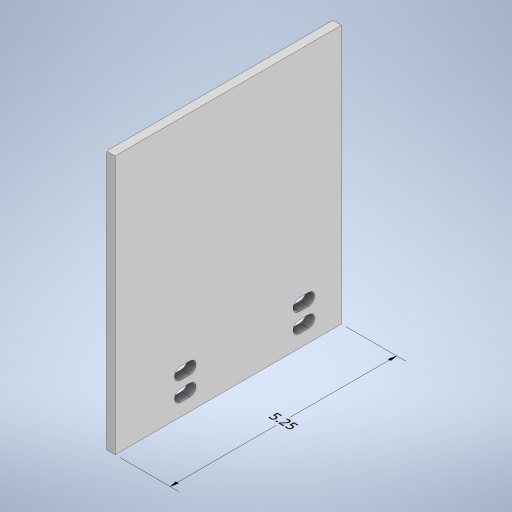
# Autodesk Inventor part: HalfFrontWall
Saved by Autodesk Inventor 2024.3 (Build 283343010, 343A)
## iProperties
Created: 2025-04-11
Part Number: HalfFrontWall
Material: Generic
Document SubType Name: Modeling
Designer: Vincent Larson
Density: 1 g/cm^3
Appearance: Default
Author: Vincent Larson
Autodesk Inventor part; units mm, degrees
ref_plane "YZ Plane" through (0, 0, 0) normal (1, 0, 0) x (0, 1, 0)
ref_plane "XZ Plane" through (0, 0, 0) normal (0, 1, 0) x (-1, 0, 0)
ref_plane "XY Plane" through (0, 0, 0) normal (0, 0, 1) x (1, 0, 0)
sketch "Sketch1" plane through (0, 0, 0) normal (0, 0, 1) x (1, 0, 0)
  point P0 (0, 0)
sketch "Sketch2" plane through (0, 0, 0) normal (1, 0, 0) x (0, 1, 0)
  line L0 (0, 0) -> (-152.4, 0)
  line L1 (-152.4, 0) -> (-152.4, -133.35)
  line L2 (-152.4, -133.35) -> (0, -133.35)
  line L3 (0, -133.35) -> (0, 0)
  dimension "d0" = 152.4
  dimension "d1" = 133.35
  constraints: 8 end point, 2 parallel, 1 horizontal, 1 perpendicular
  measures "d0" distance of L2.end L1.end
  measures "d1" distance of L1.end L0.end
extrude "Extrusion1" add sketch "Sketch2" along normal blind 5.08
sketch "Sketch6" plane through (5.08, 0, 0) normal (1, 0, 0) x (0, 0, -1)
  line L0 (0, -152.4) -> (133.35, -152.4) projected
  line L1 (133.35, -152.4) -> (133.35, 0) projected
  line L2 (0, 0) -> (0, -152.4) projected
  line L3 (41.275, -130.048) -> (47.625, -130.048)
  line L4 (47.625, -130.048) -> (41.275, -130.048)
  line L5 (41.275, -130.048) -> (34.925, -130.048)
  line L6 (34.925, -130.048) -> (47.625, -130.048) construction
  line L7 (38.4175, -133.5405) -> (44.1325, -133.5405)
  line L8 (44.1325, -126.5555) -> (38.4175, -126.5555)
  arc A0 (38.4175, -126.5555) -> (38.4175, -133.5405) centre (38.4175, -130.048) ccw
  arc A1 (44.1325, -133.5405) -> (44.1325, -126.5555) centre (44.1325, -130.048) ccw
  line L9 (111.125, -130.048) -> (117.475, -130.048)
  line L10 (117.475, -130.048) -> (111.125, -130.048)
  line L11 (111.125, -130.048) -> (104.775, -130.048)
  line L12 (104.775, -130.048) -> (117.475, -130.048) construction
  line L13 (108.2675, -133.5405) -> (113.9825, -133.5405)
  line L14 (113.9825, -126.5555) -> (108.2675, -126.5555)
  arc A2 (108.2675, -126.5555) -> (108.2675, -133.5405) centre (108.2675, -130.048) ccw
  arc A3 (113.9825, -133.5405) -> (113.9825, -126.5555) centre (113.9825, -130.048) ccw
  line L15 (41.275, -141.351) -> (47.625, -141.351)
  line L16 (47.625, -141.351) -> (41.275, -141.351)
  line L17 (41.275, -141.351) -> (34.925, -141.351)
  line L18 (34.925, -141.351) -> (47.625, -141.351) construction
  line L19 (38.4175, -144.8435) -> (44.1325, -144.8435)
  line L20 (44.1325, -137.8585) -> (38.4175, -137.8585)
  arc A4 (38.4175, -137.8585) -> (38.4175, -144.8435) centre (38.4175, -141.351) ccw
  arc A5 (44.1325, -144.8435) -> (44.1325, -137.8585) centre (44.1325, -141.351) ccw
  line L21 (111.125, -141.351) -> (117.475, -141.351)
  line L22 (111.125, -141.351) -> (104.775, -141.351)
  line L23 (104.775, -141.351) -> (117.475, -141.351) construction
  line L24 (108.2675, -144.8435) -> (113.9825, -144.8435)
  line L25 (113.9825, -137.8585) -> (108.2675, -137.8585)
  arc A6 (108.2675, -137.8585) -> (108.2675, -144.8435) centre (108.2675, -141.351) ccw
  arc A7 (113.9825, -144.8435) -> (113.9825, -137.8585) centre (113.9825, -141.351) ccw
  dimension "d28" = 6.35
  dimension "d30" = 6.985
  dimension "d31" = 6.35
  dimension "d32" = 6.35
  dimension "d33" = 6.985
  dimension "d34" = 6.35
  dimension "d35" = 6.35
  dimension "d36" = 6.985
  dimension "d37" = 6.35
  dimension "d38" = 6.35
  dimension "d39" = 6.985
  constraints: 54 end point, 24 point on circle, 16 tangent, 8 centre point, 8 point on line, 5 equal length, 4 midpoint, 1 horizontal
  measures "d28" distance of L3.start L3.end
  measures "d30" diameter of A1
  measures "d31" distance of L9.start L9.end
  measures "d32" distance of L9.start L11.end
  measures "d33" diameter of A3
  measures "d34" distance of L15.start L15.end
  measures "d35" distance of L15.start L17.end
  measures "d36" diameter of A5
  measures "d37" distance of L21.start L21.end
  measures "d38" distance of L21.start L22.end
  measures "d39" diameter of A7
extrude "Extrusion5" cut sketch "Sketch6" against normal blind 25.4
body "Solid1"
